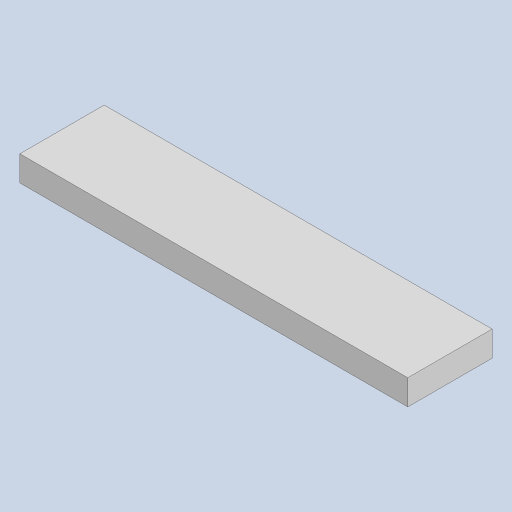
# Autodesk Inventor part: Glue holder middle block
Saved by Autodesk Inventor 2023.4 (Build 274418000, 418)
## iProperties
Created: 2023-10-31
Part Number: Glue holder middle block
Material: Generic
Document SubType Name: Modeling
Designer: PalumaCAD
Density: 1 g/cm^3
Appearance: Default
Author: PalumaCAD
Autodesk Inventor part; units mm, degrees
ref_plane "YZ Plane" through (0, 0, 0) normal (1, 0, 0) x (0, 1, 0)
ref_plane "XZ Plane" through (0, 0, 0) normal (0, 1, 0) x (-1, 0, 0)
ref_plane "XY Plane" through (0, 0, 0) normal (0, 0, 1) x (1, 0, 0)
sketch "Sketch1" plane through (0, 0, 0) normal (0, 0, 1) x (1, 0, 0)
  line L0 (-23, -1.5) -> (23, -1.5)
  line L1 (23, -1.5) -> (23, 1.5)
  line L2 (23, 1.5) -> (-23, 1.5)
  line L3 (-23, 1.5) -> (-23, -1.5)
  line L4 (-23, -1.5) -> (23, 1.5) construction
  line L5 (23, -1.5) -> (-23, 1.5) construction
  point P0 (0, 0)
  dimension "d0" = 46
  dimension "d1" = 3
  constraints: 12 end point, 2 midpoint, 2 parallel, 1 horizontal, 1 perpendicular
  measures "d0" distance of L2.end L1.end
  measures "d1" distance of L1.end L0.end
extrude "Extrusion1" add sketch "Sketch1" along normal blind 10
body "Solid1"
